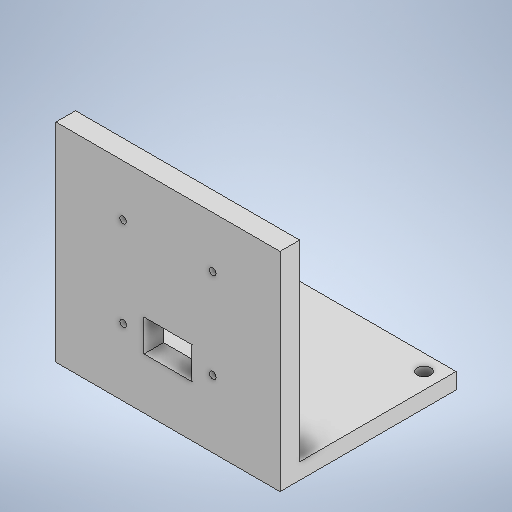
# Autodesk Inventor part: camera_bottom
Saved by Autodesk Inventor 2026.1 (Build 301233000, 233)
## iProperties
Created: 2026-05-25
Part Number: camera_bottom
Material: Generic
Document SubType Name: Modeling
Designer: chris
Density: 1 g/cm^3
Appearance: Default
Author: chris
Autodesk Inventor part; units mm, degrees
ref_plane "YZ Plane" through (0, 0, 0) normal (1, 0, 0) x (0, 1, 0)
ref_plane "XZ Plane" through (0, 0, 0) normal (0, 1, 0) x (-1, 0, 0)
ref_plane "XY Plane" through (0, 0, 0) normal (0, 0, 1) x (1, 0, 0)
sketch "Sketch1" plane through (0, 0, 0) normal (0, 1, 0) x (-1, 0, 0)
  line L0 (35, 27.5) -> (-35, 27.5)
  line L1 (-35, 27.5) -> (-35, -27.5)
  line L2 (-35, -27.5) -> (35, -27.5)
  line L3 (35, -27.5) -> (35, 27.5)
  line L4 (35, 27.5) -> (-35, -27.5) construction
  line L5 (-35, 27.5) -> (35, -27.5) construction
  point P0 (0, 0)
  dimension "d0" = 70
  dimension "d1" = 55
  constraints: 12 end point, 2 midpoint, 2 parallel, 1 horizontal, 1 perpendicular
  measures "d0" distance of L2.end L1.end
  measures "d1" distance of L1.end L0.end
extrude "Extrusion1" add sketch "Sketch1" along normal blind 5
sketch "Sketch2" plane through (0, 5, 0) normal (0, 1, 0) x (1, 0, 0)
  circle A0 centre (-30, 22.5) radius 2.1
  circle A1 centre (30, 22.5) radius 2.1
  line L0 (35, 27.5) -> (-35, 27.5) projected
  line L1 (-35, 27.5) -> (-35, -27.5) projected
  line L2 (35, -27.5) -> (35, 27.5) projected
  point P0 (0, 0)
  dimension "d4" = 4.2
  dimension "d5" = 4.2
  dimension "d6" = 5
  dimension "d7" = 5
  dimension "d8" = 5
  dimension "d9" = 5
  constraints: 2 centre point
  measures "d4" diameter of A0
  measures "d5" diameter of A1
  measures "d6" distance from line of L0 A0.centre
  measures "d7" distance from line of L1 A0.centre
  measures "d8" distance from line of L0 A1.centre
  measures "d9" distance from line of L2 A1.centre
extrude "Extrusion2" cut sketch "Sketch2" against normal blind 5
sketch "Sketch3" plane through (0, 5, 0) normal (0, 1, 0) x (1, 0, 0)
  line L0 (-35, -27.5) -> (35, -27.5)
  line L1 (35, -27.5) -> (35, -21.3758)
  line L2 (35, -21.3758) -> (-35, -21.3758)
  line L3 (-35, -21.3758) -> (-35, -27.5)
  line L4 (-35, -27.5) -> (35, -21.3758) construction
  line L5 (35, -27.5) -> (-35, -21.3758) construction
  line L6 (-35, -27.5) -> (35, -27.5) projected
  line L7 (35, -27.5) -> (35, 27.5) projected
  line L8 (-35, 27.5) -> (-35, -27.5) projected
  point P0 (0, 0)
  point P1 (0, -24.4379)
  dimension "d12" = 5
  constraints: 12 end point, 3 collinear, 2 midpoint, 2 parallel, 1 horizontal, 1 perpendicular
  measures "d12" angle of L5 L2
extrude "Extrusion3" add sketch "Sketch3" along normal blind 60
sketch "Sketch4" plane through (-35, 0, 27.5) normal (0, 0, 1) x (1, 0, 0)
  circle A0 centre (21, 49) radius 1.05
  circle A1 centre (49, 49) radius 1.05
  circle A2 centre (21, 21) radius 1.05
  circle A3 centre (49, 21) radius 1.05
  line L0 (0, 0) -> (70, 0) projected
  line L1 (70, 0) -> (70, 65) projected
  line L2 (0, 0) -> (0, 65) projected
  point P0 (35, 0)
  dimension "d15" = 2.1
  dimension "d16" = 2.1
  dimension "d17" = 2.1
  dimension "d18" = 2.1
  dimension "d19" = 21
  dimension "d20" = 21
  dimension "d21" = 21
  dimension "d22" = 28
  constraints: 4 centre point, 2 horizontal alignment, 2 vertical alignment
  measures "d15" diameter of A0
  measures "d16" diameter of A1
  measures "d17" diameter of A2
  measures "d18" diameter of A3
  measures "d19" distance from line of L1 A3.centre
  measures "d20" distance from line of L2 A2.centre
  measures "d21" distance from line of L0 A3.centre
  measures "d22" distance of A3.centre A1.centre
extrude "Extrusion4" cut sketch "Sketch4" against normal blind 50
sketch "Sketch5" plane through (-35, 0, 27.5) normal (0, 0, 1) x (1, 0, 0)
  line L0 (27.5, 16) -> (42.5, 16)
  line L1 (42.5, 16) -> (42.5, 26)
  line L2 (42.5, 26) -> (27.5, 26)
  line L3 (27.5, 26) -> (27.5, 16)
  line L4 (27.5, 16) -> (42.5, 26) construction
  line L5 (42.5, 16) -> (27.5, 26) construction
  line L6 (0, 0) -> (70, 0) projected
  point P0 (35, 0)
  point P1 (35, 21)
  point P2 (35, 0)
  dimension "d25" = 15
  dimension "d26" = 10
  dimension "d27" = 21
  constraints: 12 end point, 3 midpoint, 2 parallel, 1 horizontal, 1 perpendicular
  measures "d25" distance of L2.end L1.end
  measures "d26" distance of L0.end L1.end
  measures "d27" distance of point (35, 0) point (35, 21)
extrude "Extrusion5" cut sketch "Sketch5" against normal blind 50
body "Solid1"
